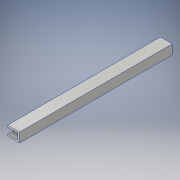
# Autodesk Inventor part: 1 x 16 x 3_16
Saved by Autodesk Inventor 2016 (Build 200138000, 138)
## iProperties
Created: 2015-06-18
Part Number: 1 x 16 x 3_16
Material: Aluminum 6061
Document SubType Name: Modeling
Designer: steele
Density: 2.7 g/cm^3
Appearance: Aluminum - Flat
Mass: 414.798 g
Surface Area: 691.43 cm^2
Volume: 153.629 cm^3
Author: steele
Autodesk Inventor part; units mm, degrees
ref_plane "YZ Plane" through (0, 0, 0) normal (1, 0, 0) x (0, 1, 0)
ref_plane "XZ Plane" through (0, 0, 0) normal (0, 1, 0) x (-1, 0, 0)
ref_plane "XY Plane" through (0, 0, 0) normal (0, 0, 1) x (1, 0, 0)
sketch "Sketch1" plane through (0, 0, 0) normal (0, 0, 1) x (1, 0, 0)
  line L0 (0, 0) -> (0, 12.7)
  line L1 (0, 12.7) -> (-31.75, 12.7)
  line L2 (-31.75, 12.7) -> (-31.75, 7.9375)
  line L3 (-31.75, 7.9375) -> (-4.7625, 7.9375)
  line L4 (-4.7625, 7.9375) -> (-4.7625, 0)
  line L5 (0, 0) -> (0, -12.7)
  line L6 (0, -12.7) -> (-31.75, -12.7)
  line L7 (-31.75, -12.7) -> (-31.75, -7.9375)
  line L8 (-31.75, -7.9375) -> (-4.7625, -7.9375)
  line L9 (-4.7625, -7.9375) -> (-4.7625, 0)
  dimension "width" = 25.4
  dimension "thickness" = 4.7625
  dimension "d2" = 4.7625
  dimension "height" = 31.75
  constraints: 20 end point, 4 perpendicular, 3 collinear, 1 vertical
  measures "width" distance between parallel lines of L6 L1
  measures "thickness" distance between parallel lines of L4 L0
  measures "d2" distance between parallel lines of L3 L1
  measures "height" distance between parallel lines of L0 L2
extrude "Extrusion1" add sketch "Sketch1" along normal mid plane 406.4
equation "\"d2\" = thickness"
body "Solid1"
